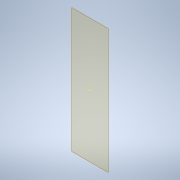
# Autodesk Inventor part: silla
Saved by Autodesk Inventor 2021 (Build 250183000, 183)
## iProperties
Created: 2021-03-18
Part Number: silla
Material: Lead
Document SubType Name: Modeling
Designer: andre
Density: 11.34 g/cm^3
Appearance: Lead
Author: andre
Autodesk Inventor part; units mm, degrees
ref_plane "YZ Plane" through (0, 0, 0) normal (1, 0, 0) x (0, 1, 0)
ref_plane "XZ Plane" through (0, 0, 0) normal (0, 1, 0) x (-1, 0, 0)
ref_plane "XY Plane" through (0, 0, 0) normal (0, 0, 1) x (1, 0, 0)
ref_plane "Work Plane1" through (0, 0, 0) normal (0, 0, 1) x (1, 0, 0)
sketch "Sketch1" plane through (0, 0, 0) normal (0, 0, 1) x (1, 0, 0)
  circle A0 centre (143.9667, 339.6714) radius 113.8379
  line L0 (-337.5, 1050) -> (337.5, 1050)
  line L1 (-337.5, 600) -> (337.5, 600)
  line L2 (337.5, 600) -> (337.5, 1050)
  line L3 (337.5, 1050) -> (-337.5, 1050)
  line L4 (-337.5, 1050) -> (-337.5, 600)
  point P0 (0, 0)
  constraints: 10 end point, 2 horizontal, 2 parallel, 1 centre point, 1 perpendicular, 3 other
extrude "Extrusion1" add sketch "Sketch1" along normal blind 150 contours L0 L2 L1 L4
sketch "Sketch2" plane through (0, 0, 150) normal (0, 0, 1) x (1, 0, 0)
  line L0 (-337.5, 600) -> (337.5, 600) projected
  line L1 (337.5, 1050) -> (-337.5, 1050) projected
  line L2 (337.5, 600) -> (237.5, 600)
  line L3 (237.5, 600) -> (237.5, 1050)
  line L4 (237.5, 1050) -> (337.5, 1050)
  line L5 (337.5, 1050) -> (337.5, 600)
  point P0 (0, 0)
  point P1 (237.5, 600)
  dimension "d2" = 100
  constraints: 8 end point, 2 parallel, 1 horizontal, 1 perpendicular, 1 point on line
  measures "d2" distance between parallel lines of L5 L3
extrude "Extrusion2" add sketch "Sketch2" along normal blind 700
body "Solid1"
